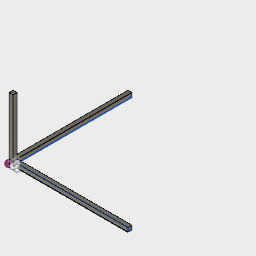
Kalibrierwinkel Outline 5mm 145x145x75mm v3 v2 (Autodesk Fusion 360 design; units mm, degrees)
Autodesk Fusion 360 part; units mm, degrees
sketch "Skizze1" plane through (0, 0, 0) normal (0, 0, 1) x (1, 0, 0)
  line L0 (0, 0) -> (145, 0)
  line L1 (0, 145) -> (0, 0)
  line L2 (0, 0) -> (10, 0)
  line L3 (0, 10) -> (0, 0)
  line L4 (5, 145) -> (5, 5)
  line L5 (5, 145) -> (0, 145)
  line L6 (145, 0) -> (145, 5)
  line L7 (145, 5) -> (0, 5)
  line L8 (5, 0) -> (5, 5)
extrude "Extrusion11" add sketch "Skizze1" along normal blind 75 contours L0 L1 L2 L3 L7 L8 makes body 1
extrude "Extrusion12" add sketch "Skizze1" along normal blind 5 separate body makes body 2
